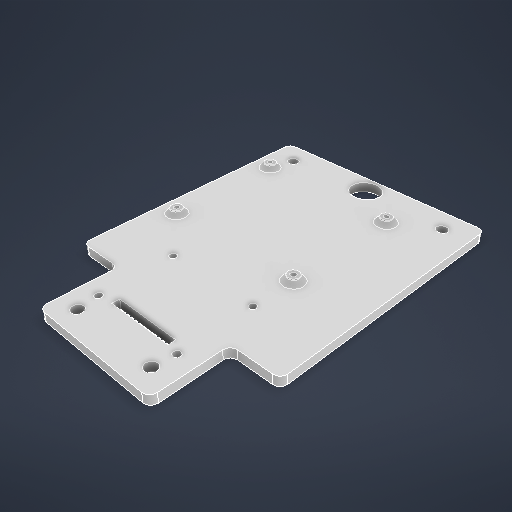
# Autodesk Inventor part: 1.5_base_2
Saved by Autodesk Inventor 2025 (Build 290162000, 162)
## iProperties
Created: 2024-05-22
Part Number: 1.5_base_2
Material: Generic
Document SubType Name: Modeling
Designer: Garfieldcmix
Density: 1 g/cm^3
Appearance: Default
Author: Garfieldcmix
Autodesk Inventor part; units mm, degrees
ref_plane "YZ Plane" through (0, 0, 0) normal (1, 0, 0) x (0, 1, 0)
ref_plane "XZ Plane" through (0, 0, 0) normal (0, 1, 0) x (-1, 0, 0)
ref_plane "XY Plane" through (0, 0, 0) normal (0, 0, 1) x (1, 0, 0)
derived "Car_Plan.ipt"
sketch "Car_Sketch" plane through (0, 0, 0) normal (0, 1, 0) x (-1, 0, 0)
  line L0 (0, 0) -> (94, 0)
  line L1 (0, 0) -> (0, 105)
  line L2 (94, 0) -> (94, 105)
  line L3 (0, 105) -> (20, 105)
  line L4 (20, 105) -> (20, 190)
  line L5 (20, 190) -> (74, 190)
  line L6 (74, 190) -> (74, 105)
  line L7 (74, 105) -> (94, 105)
  line L8 (-5, 68) -> (-5, 0)
  line L9 (-5, 0) -> (-32, 0)
  line L10 (-32, 0) -> (-32, 68)
  line L11 (-32, 68) -> (-5, 68)
  line L12 (47, 190) -> (47, 0) construction
  line L13 (126, 68) -> (99, 68)
  line L14 (99, 68) -> (99, 0)
  line L15 (126, 0) -> (126, 68)
  line L16 (99, 0) -> (126, 0)
  line L17 (-5, 34) -> (99, 34) construction
  line L18 (0, 95) -> (94, 95) construction
  line L19 (-5, 190) -> (-32, 190)
  line L20 (-32, 122) -> (-5, 122)
  line L21 (-32, 190) -> (-32, 122)
  line L22 (-5, 122) -> (-5, 190)
  line L23 (-5, 156) -> (99, 156) construction
  line L24 (126, 122) -> (99, 122)
  line L25 (126, 190) -> (126, 122)
  line L26 (99, 190) -> (126, 190)
  line L27 (99, 122) -> (99, 190)
  line L28 (0, 156) -> (47, 34) construction
  line L29 (94, 156) -> (47, 34) construction
  line L30 (0, 156) -> (-174.2341, 34) construction
  line L31 (-5, 34) -> (-174.2341, 34) construction
  line L32 (8.9873, 132.6713) -> (47, 142.55) construction
  line L33 (85.0127, 132.6713) -> (47, 142.55) construction
  line L34 (0, 102) -> (-12, 102)
  line L35 (-12, 102) -> (-12, 78)
  line L36 (-12, 78) -> (0, 78)
  line L37 (106, 78) -> (94, 78)
  line L38 (106, 102) -> (106, 78)
  line L39 (94, 102) -> (106, 102)
sketch "Base" plane through (0, 0, 0) normal (0, 1, 0) x (-1, 0, 0)
  line L0 (0, 0) -> (0, 105) projected
  line L1 (0, 105) -> (20, 105) projected
  line L2 (20, 105) -> (20, 190) projected
  line L3 (74, 190) -> (74, 105) projected
  line L4 (74, 105) -> (94, 105) projected
  line L5 (94, 0) -> (94, 105) projected
  line L6 (0, 0) -> (94, 0) projected
  line L7 (74, 135) -> (20, 135)
  circle A0 centre (29, 127) radius 2.4
  circle A1 centre (65, 127) radius 2.4
  circle A2 centre (11.1, 10) radius 2.4
  circle A3 centre (82.9, 10) radius 2.4
  dimension "d76" = 30
  dimension "d77" = 4.8
  dimension "d78" = 4.8
  dimension "d79" = 9
  dimension "d80" = 22
  dimension "d81" = 22
  dimension "d82" = 9
  dimension "d83" = 4.8
  dimension "d84" = 4.8
  dimension "d85" = 10
  dimension "d86" = 11.1
  dimension "d87" = 10
  dimension "d88" = 11.1
  constraints: 4 centre point, 2 end point, 2 point on line, 1 perpendicular
  measures "d76" distance between parallel lines of L1 L7
  measures "d77" diameter of A0
  measures "d78" diameter of A1
  measures "d79" distance from line of L2 A0.centre
  measures "d80" distance from line of L1 A0.centre
  measures "d81" distance from line of A1.centre L4
  measures "d82" distance from line of L3 A1.centre
  measures "d83" diameter of A2
  measures "d84" diameter of A3
  measures "d85" distance from line of L6 A2.centre
  measures "d86" distance from line of L0 A2.centre
  measures "d87" distance from line of L6 A3.centre
  measures "d88" distance from line of L5 A3.centre
extrude "Extrusion1" add sketch "Base" along normal blind 4
fillet "Fillet2" radius 3 8 edges at (-20, 2, 105) (0, 2, 105) (0, 2, 0) (-94, 2, 0) (-94, 2, 105) (-74, 2, 105) (-74, 2, 135) (-20, 2, 135)
sketch "Raspi_Sketch" plane through (0, 4, 0) normal (0, 1, 0) x (1, 0, 0)
  line L0 (0, -102) -> (0, -3) projected
  line L1 (-17, -105) -> (-3, -105) projected
  line L2 (-94, -3) -> (-94, -102) projected
  line L3 (-91, -105) -> (-77, -105) projected
  line L4 (0, -73) -> (-4.5, -73)
  line L5 (-4.5, -73) -> (-89.5, -73)
  line L6 (-89.5, -73) -> (-89.5, -17)
  line L7 (-89.5, -17) -> (-4.5, -17)
  line L8 (-4.5, -17) -> (-4.5, -73)
  line L9 (-4.5, -73) -> (-8, -73)
  line L10 (-4.5, -69.5) -> (-4.5, -73)
  circle A0 centre (-28, -69.5) radius 1.25
  line L11 (-28, -69.5) -> (-24.5, -69.5)
  line L12 (-24.5, -69.5) -> (-24.5, -73)
  line L13 (-24.5, -73) -> (-28, -73)
  line L14 (-28, -73) -> (-28, -69.5)
  line L15 (-24.5, -73) -> (-89.5, -73)
  line L16 (-89.5, -73) -> (-89.5, -17)
  line L17 (-89.5, -17) -> (-24.5, -17)
  line L18 (-24.5, -17) -> (-24.5, -73)
  line L19 (-57, -73) -> (-57, -59.7745)
  line L20 (-24.5, -45) -> (-39.3063, -45)
  circle A1 centre (-86, -69.5) radius 1.25
  circle A2 centre (-28, -20.5) radius 1.25
  circle A3 centre (-86, -20.5) radius 1.25
  circle A4 centre (-28, -69.5) radius 2.5
  circle A5 centre (-86, -69.5) radius 2.5
  circle A6 centre (-28, -20.5) radius 2.5
  circle A7 centre (-86, -20.5) radius 2.5
  point P0 (0, 0)
  dimension "d196" = 4.5
  dimension "d197" = 85
  dimension "d198" = 56
  dimension "d199" = 32
  dimension "d202" = 2.5
  dimension "d203" = 3.5
  dimension "d204" = 23.5
  dimension "d205" = 3.5
  dimension "d242" = 5
  constraints: 34 end point, 8 centre point, 6 horizontal, 6 parallel, 6 symmetric about line, 3 perpendicular, 2 midpoint, 2 point on line, 1 coincident, 1 vertical, 6 other
  measures "d196" distance of L4.start L4.end
  measures "d197" distance of L6.end L7.end
  measures "d198" distance of L5.end L6.end
  measures "d199" distance between parallel lines of L1 L4
  measures "d202" diameter of A0
  measures "d203" distance from line of L5 L11.start
  measures "d204" distance from line of L8 L11.start
  measures "d205" distance of L12.end L13.end
  measures "d242" diameter of A4
extrude "Raspi_Hole" cut sketch "Raspi_Sketch" against normal through all contours L14 L11 A0 | A0 L11 L14 | A1 | A2 | A3
extrude "Raspi_Extrude" add sketch "Raspi_Sketch" along normal blind 2.5 contours A4 L11 A0 L14 | L14 A0 L11 A4 | A5 | A6 | A7
sketch "Sketch22" plane through (0, 4, 0) normal (0, 1, 0) x (1, 0, 0)
  line L0 (-3, 0) -> (-91, 0) construction
  line L1 (-47, 0) -> (-47, -8) construction
  circle A0 centre (-47, -8) radius 6.5
  point P0 (0, 0)
  dimension "d249" = 8
  dimension "d250" = 13
  constraints: 2 end point, 1 centre point, 1 coincident, 1 midpoint, 1 perpendicular
  measures "d249" distance of L1.start L1.end
  measures "d250" diameter of A0
extrude "Extrusion16" cut sketch "Sketch22" against normal through all
sketch "Sketch20" plane through (0, 4, 0) normal (0, 1, 0) x (1, 0, 0)
  line L0 (0, -102) -> (0, -3) projected
  line L1 (-3, 0) -> (-91, 0) projected
  line L2 (-25.41, -85.44) -> (-68.59, -85.44)
  line L3 (-68.59, -85.44) -> (-68.59, -121)
  line L4 (-68.59, -121) -> (-25.41, -121)
  line L5 (-25.41, -121) -> (-25.41, -85.44)
  line L6 (-25.41, -121) -> (-27.94, -121)
  line L7 (-25.41, -118.46) -> (-25.41, -121)
  circle A0 centre (-27.95, -118.46) radius 1.5
  line L8 (-68.59, -85.44) -> (-52.5718, -85.44)
  line L9 (-59.89, -114.8) -> (-32.89, -114.8)
  line L10 (-32.89, -114.8) -> (-32.89, -117.8)
  line L11 (-32.89, -117.8) -> (-59.89, -117.8)
  line L12 (-59.89, -117.8) -> (-59.89, -114.8)
  line L13 (-68.59, -103.22) -> (-25.41, -103.22) construction
  line L14 (-47, -121) -> (-47, -85.44) construction
  circle A1 centre (-66.05, -118.46) radius 1.5
  circle A2 centre (-27.95, -87.98) radius 1.5
  circle A3 centre (-66.05, -87.98) radius 1.5
  line L15 (-71, -135) -> (-23, -135) construction
  line L16 (-47, -135) -> (-47, -121) construction
  point P0 (0, 0)
  dimension "d210" = 43.18
  dimension "d211" = 35.56
  dimension "d214" = 3
  dimension "d233" = 27
  dimension "d234" = 3
  dimension "d237" = 8.7
  dimension "d238" = 3.2
  dimension "d239" = 2.54
  dimension "d240" = 2.54
  dimension "d241" = 14
  constraints: 28 end point, 5 midpoint, 4 centre point, 4 horizontal, 4 parallel, 3 perpendicular, 3 symmetric about line, 3 other
  measures "d210" distance of L4.end L3.end
  measures "d211" distance of L3.end L2.end
  measures "d214" diameter of A0
  measures "d233" distance of L10.end L11.end
  measures "d234" distance of L9.end L10.end
  measures "d237" distance from line of L3 L11.end
  measures "d238" distance from line of L4 L11.end
  measures "d239" distance from line of L5 A0.centre
  measures "d240" distance from line of L4 A0.centre
  measures "d241" distance between parallel lines of L4 L15
extrude "Maker_Drive_Holder" cut sketch "Sketch20" against normal through all contours A0 | L9 L10 L11 L12 | A1 | A2 | A3
chamfer "Chamfer1" distance 2 angle 45 4 edges at (-30.5, 4, 69.5) (-88.5, 4, 69.5) (-30.5, 4, 20.5) (-88.5, 4, 20.5)
body "Solid1"
